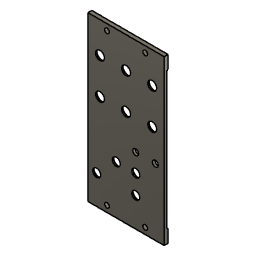
CHORDS Module Faceplate Generator (Autodesk Fusion 360 design; units mm, degrees)
Autodesk Fusion 360 part; units mm, degrees
note: some values were not read from the file. Chosen so that the rebuilt part matches the saved one: which face or edge a step refers to. Set by a fixed rule: which sketch regions a step uses.
(part 1 of 2)
sketch "Sketch2" plane through (0, 0, 0) normal (0, 0, 1) x (1, 0, 0)
  line L0 (29.9, 50) -> (-29.9, 50)
  line L1 (-29.9, 50) -> (-29.9, -50)
  line L2 (-29.9, -50) -> (29.9, -50)
  line L3 (29.9, -50) -> (29.9, 50)
  line L4 (29.9, 50) -> (-29.9, -50) construction
  line L5 (-29.9, 50) -> (29.9, -50) construction
  circle A0 centre (-20.5, 44) radius 4 construction
  circle A1 centre (0, 44) radius 4 construction
  circle A2 centre (20.5, 44) radius 4 construction
  circle A3 centre (-20.5, 16) radius 4 construction
  circle A4 centre (0, 16) radius 4 construction
  circle A5 centre (20.5, 16) radius 4 construction
  circle A6 centre (7.5858, -21.8615) radius 4 construction
  circle A7 centre (22.8605, -21.6215) radius 4 construction
  circle A8 centre (-23.0435, -21.8245) radius 4 construction
  circle A9 centre (-7.6771, -21.8488) radius 4 construction
  circle A10 centre (-23.0823, -36.9623) radius 4 construction
  circle A11 centre (-7.7159, -36.9866) radius 4 construction
  circle A12 centre (7.547, -36.9993) radius 4 construction
  circle A13 centre (22.8217, -36.7594) radius 4 construction
  line L6 (29.9, 50) -> (-29.9, 50)
  line L7 (29.9, -50) -> (-29.9, -50)
  line L8 (-29.9, -50) -> (-29.9, -59.9)
  line L9 (-29.9, -59.9) -> (29.9, -59.9)
  line L10 (29.9, -59.9) -> (29.9, -50)
  circle A14 centre (22.9516, -7.7584) radius 3 construction
  circle A15 centre (7.5143, -7.6767) radius 3 construction
  circle A16 centre (20.5, 16) radius 3.5
  circle A17 centre (20.5, 44) radius 3.5
  circle A18 centre (0, 44) radius 3.5
  circle A19 centre (-20.5, 44) radius 3.5
  circle A20 centre (-20.5, 16) radius 3.5
  circle A21 centre (0, 16) radius 3.5
  line L11 (29.9, 50) -> (-29.9, 50)
  line L12 (-29.9, 50) -> (-29.9, 68.4)
  line L13 (-29.9, 68.4) -> (29.9, 68.4)
  line L14 (29.9, 68.4) -> (29.9, 50)
  circle A22 centre (22.8605, -21.6215) radius 3.15
  circle A23 through (7.5858, -18.7115, 0) (7.5858, -23.4365, 2.728) (7.5858, -23.4365, -2.728) construction
  circle A24 centre (7.5858, -21.8615) radius 3.15
  circle A25 centre (-7.6771, -21.8488) radius 3.15
  circle A26 centre (-23.0435, -21.8245) radius 3.15
  circle A27 centre (22.8217, -36.7594) radius 3.15
  circle A28 centre (7.547, -36.9993) radius 3.15
  circle A29 centre (-7.7159, -36.9866) radius 3.15
  circle A30 centre (-23.0823, -36.9623) radius 3.15
  circle A31 centre (22.9516, -7.7584) radius 2.325
  circle A32 centre (7.5143, -7.6767) radius 2.325
  line L15 (0, 12.5) -> (0, 9.3) construction
  line L16 (0, 9.3) -> (-29.9, 9.3) construction
  line L17 (0, 9.3) -> (29.9, 9.3) construction
  line L18 (0, 9.3) -> (-1, 9.3) construction
  line L19 (-1, 9.3) -> (1, 9.3)
  line L20 (1, 9.3) -> (1, 11.3)
  line L21 (1, 11.3) -> (-1, 11.3)
  line L22 (-1, 11.3) -> (-1, 9.3)
  line L23 (0, 40.5) -> (0, 37.3) construction
  line L24 (0, 37.3) -> (-29.9, 37.3) construction
  line L25 (0, 37.3) -> (29.9, 37.3) construction
  line L26 (0, 37.3) -> (-1, 37.3) construction
  line L27 (-1, 37.3) -> (1, 37.3)
  line L28 (1, 37.3) -> (1, 39.3)
  line L29 (1, 39.3) -> (-1, 39.3)
  line L30 (-1, 39.3) -> (-1, 37.3)
  line L31 (20.5, 44) -> (20.5, 9.3) construction
  line L32 (20.5, 37.3) -> (19.5, 37.3) construction
  line L33 (19.5, 37.3) -> (19.5, 9.3) construction
  line L34 (19.5, 9.3) -> (21.5, 9.3)
  line L35 (21.5, 9.3) -> (21.5, 11.3)
  line L36 (21.5, 11.3) -> (19.5, 11.3)
  line L37 (19.5, 11.3) -> (19.5, 9.3)
  line L38 (19.5, 37.3) -> (21.5, 37.3)
  line L39 (21.5, 37.3) -> (21.5, 39.3)
  line L40 (21.5, 39.3) -> (19.5, 39.3)
  line L41 (19.5, 39.3) -> (19.5, 37.3)
  line L42 (-20.5, 44) -> (-20.5, 9.3) construction
  line L43 (-20.5, 37.3) -> (-21.5, 37.3) construction
  line L44 (-21.5, 37.3) -> (-19.5, 37.3)
  line L45 (-19.5, 37.3) -> (-19.5, 39.3)
  line L46 (-19.5, 39.3) -> (-21.5, 39.3)
  line L47 (-21.5, 39.3) -> (-21.5, 37.3)
  line L48 (-21.5, 9.3) -> (-19.5, 9.3)
  line L49 (-19.5, 9.3) -> (-19.5, 11.3)
  line L50 (-19.5, 11.3) -> (-21.5, 11.3)
  line L51 (-21.5, 11.3) -> (-21.5, 9.3)
  dimension "d1" = 59.8
  dimension "d2" = 100
  dimension "d3" = 8
  dimension "d4" = 8
  dimension "d5" = 8
  dimension "d6" = 8
  dimension "d7" = 8
  dimension "d8" = 8
  dimension "d9" = 8
  dimension "d10" = 8
  dimension "d11" = 8
  dimension "d12" = 8
  dimension "d13" = 8
  dimension "d14" = 8
  dimension "d15" = 8
  dimension "d16" = 8
  dimension "d18" = 9.9
  dimension "d25" = 6
  dimension "d26" = 6
  dimension "d29" = 7
  dimension "d30" = 7
  dimension "d31" = 7
  dimension "d32" = 7
  dimension "d33" = 7
  dimension "d34" = 7
  dimension "d36" = 18.4
  dimension "d37" = 6.3
  dimension "d38" = 6.3
  dimension "d39" = 6.3
  dimension "d40" = 6.3
  dimension "d41" = 6.3
  dimension "d42" = 6.3
  dimension "d43" = 6.3
  dimension "d44" = 6.3
  dimension "d45" = 6.3
  dimension "d47" = 4.65
  dimension "d48" = 4.65
  dimension "d56" = 3.2
  dimension "d57" = 1
  dimension "d58" = 2
  dimension "d59" = 2
  dimension "d60" = 3.2
  dimension "d61" = 1
  dimension "d62" = 2
  dimension "d63" = 2
  dimension "d64" = 1
  dimension "d65" = 2
  dimension "d66" = 2
  dimension "d67" = 2
  dimension "d68" = 2
  dimension "d69" = 1
  dimension "d70" = 2
  dimension "d71" = 2
  dimension "d72" = 2
  dimension "d73" = 2
  constraint horizontal L0
  constraint perpendicular L0 L1
  constraint parallel L0 L2
  constraint parallel L1 L3
  constraint coincident L4 origin
  constraint coincident L5 origin
  constraint horizontal L6
  constraint horizontal L7
  constraint vertical L8
  constraint horizontal L9
  constraint vertical L10
  constraint concentric A5 A16
  constraint concentric A2 A17
  constraint concentric A1 A18
  constraint concentric A0 A19
  constraint concentric A3 A20
  constraint concentric A4 A21
  constraint horizontal L11
  constraint vertical L12
  constraint horizontal L13
  constraint vertical L14
  constraint concentric A7 A22
  constraint concentric A6 A24
  constraint concentric A9 A25
  constraint concentric A8 A26
  constraint concentric A13 A27
  constraint concentric A12 A28
  constraint concentric A11 A29
  constraint concentric A10 A30
  constraint concentric A14 A31
  constraint concentric A15 A32
  constraint coincident A21 L15.start
  constraint vertical L15
  constraint coincident L1 L16.end
  constraint perpendicular L1 L16
  constraint coincident L3 L17.end
  constraint perpendicular L3 L17
  constraint perpendicular L15 L18
  constraint horizontal L19
  constraint vertical L20
  constraint horizontal L21
  constraint vertical L22
  constraint coincident A18 L23.start
  constraint vertical L23
  constraint coincident L1 L24.end
  constraint perpendicular L1 L24
  constraint coincident L3 L25.end
  constraint perpendicular L3 L25
  constraint perpendicular L23 L26
  constraint horizontal L27
  constraint vertical L28
  constraint horizontal L29
  constraint vertical L30
  constraint coincident A2.centre A17.centre
  constraint coincident L17 L31.end
  constraint perpendicular L17 L31
  constraint coincident L31 L32.start
  constraint coincident L25 L32.start
  constraint coincident L25 L32.end
  constraint coincident L17 L33.end
  constraint perpendicular L17 L33
  constraint horizontal L34
  constraint vertical L35
  constraint horizontal L36
  constraint vertical L37
  constraint horizontal L38
  constraint vertical L39
  constraint horizontal L40
  constraint vertical L41
  constraint coincident A0.centre A19.centre
  constraint coincident L16 L42.end
  constraint perpendicular L16 L42
  constraint coincident L24 L43.start
  constraint coincident L42 L43.start
  constraint perpendicular L42 L43
  constraint horizontal L44
  constraint vertical L45
  constraint horizontal L46
  constraint vertical L47
  constraint horizontal L48
  constraint vertical L49
  constraint horizontal L50
  constraint vertical L51
  constraint coincident L16 L48.start
  constraint coincident L1.end L2.start
  constraint coincident L0.end L12
  constraint coincident L0.end L1.start
  measures "d1" distance of L1.end L2.end
  measures "d2" distance of L0.end L1.end
  measures "d3" diameter of A0
  measures "d4" diameter of A1
  measures "d5" diameter of A2
  measures "d6" diameter of A3
  measures "d7" diameter of A4
  measures "d8" diameter of A5
  measures "d9" diameter of A6
  measures "d10" diameter of A7
  measures "d11" diameter of A8
  measures "d12" diameter of A9
  measures "d13" diameter of A12
  measures "d14" diameter of A13
  measures "d15" diameter of A10
  measures "d16" diameter of A11
  measures "d18" distance of L2.end L9.end
  measures "d25" diameter of A14
  measures "d26" diameter of A15
  measures "d29" diameter of A16
  measures "d30" diameter of A17
  measures "d31" diameter of A18
  measures "d32" diameter of A19
  measures "d33" diameter of A20
  measures "d34" diameter of A21
  measures "d36" distance of L0.start L13.end
  measures "d37" diameter of A22
  measures "d39" diameter of A24
  measures "d40" diameter of A25
  measures "d41" diameter of A26
  measures "d42" diameter of A27
  measures "d43" diameter of A28
  measures "d44" diameter of A29
  measures "d45" diameter of A30
  measures "d47" diameter of A31
  measures "d48" diameter of A32
  measures "d56" distance of L15.start L15.end
  measures "d57" distance of L15.end L18.end
  measures "d58" distance of L18.end L19.end
  measures "d59" distance of L18.end L21.end
  measures "d60" distance of L23.start L23.end
  measures "d61" distance of L23.end L26.end
  measures "d62" distance of L26.end L27.end
  measures "d63" distance of L26.end L29.end
  measures "d64" distance of L32.start L32.end
  measures "d65" distance of L33.end L34.end
  measures "d66" distance of L33.end L36.end
  measures "d67" distance of L32.end L38.end
  measures "d68" distance of L32.end L40.end
  measures "d69" distance of L43.start L43.end
  measures "d70" distance of L43.end L44.end
  measures "d71" distance of L43.end L46.end
  measures "d72" distance of L48.start L48.end
  measures "d73" distance of L48.start L50.end
extrude "Extrude2" add sketch "Sketch2" along normal blind 2 contours L0 L1 L2 L3 L6 L7 L11 | L0 L6 L11 L12 L13 L14 | L2 L7 L8 L9 L10 | A22 | A26 | A27 | A29 | L19 L20 L21 L22 | L27 L28 L29 L30 | L34 L35 L36 L37 | L38 L39 L40 L41 | L44 L45 L46 L47 | L48 L49 L50 L51
extrude "Extrude3" cut sketch "Sketch2" along normal blind 1.2 contours L19 L20 L21 L22 | L27 L28 L29 L30 | L34 L35 L36 L37 | L38 L39 L40 L41 | L44 L45 L46 L47 | L48 L49 L50 L51
chamfer "Chamfer1" distance 1 angle 45 4 edges at (-26.2323, -36.9623, 0) (-10.8271, -21.8488, 0) (4.397, -36.9993, 0) (4.4358, -21.8615, 0)
chamfer "Chamfer2" distance 1 angle 45 6 edges at (17.2369, 45.2657, 0) (17.2369, 17.2657, 0) (-3.2631, 17.2657, 0) (-23.7631, 17.2657, 0) (-23.7631, 45.2657, 0) (-3.2631, 45.2657, 0)
move_face "OffsetFaces3" offset -0.3 6 faces at (20.1667, 37.3, 0.4) (-0.3333, 37.3, 0.4) (-20.8333, 37.3, 0.4) (-20.8333, 9.3, 0.4) (-0.3333, 9.3, 0.4) (20.1667, 9.3, 0.4)
move_face "OffsetFaces4" offset -0.3 6 faces at (20.8333, 39.3, 0.4) (0.3333, 39.3, 0.4) (-20.1667, 39.3, 0.4) (-20.1667, 11.3, 0.4) (0.3333, 11.3, 0.4) (20.8333, 11.3, 0.4)
move_face "OffsetFaces5" offset -0.2 6 faces at (19.5, 37.8667, 0.8) (-1, 37.8667, 0.8) (-21.5, 37.8667, 0.8) (-21.5, 9.8667, 0.8) (-1, 9.8667, 0.8) (19.5, 9.8667, 0.8)
move_face "OffsetFaces6" offset -0.2 6 faces at (21.5, 38.7333, 0.8) (21.5, 9.8667, 0.4) (1, 9.8667, 0.4) (1, 37.8667, 0.4) (-19.5, 37.8667, 0.4) (-19.5, 9.8667, 0.4)
move_face "OffsetFaces7" offset 0.5 2 faces at (9.8364, -7.5608, 0.6667) (25.2737, -7.6425, 0.6667)
sketch "Sketch5" plane through (0, 0, 2) normal (0, 0, 1) x (1, 0, 0)
  circle A0 centre (7.5858, -21.8615) radius 3.15
  circle A1 centre (-7.6771, -21.8488) radius 3.15
  circle A2 centre (22.9516, -7.7584) radius 1.825
  circle A3 centre (7.5143, -7.6767) radius 1.825
  line L0 (-29.9, 68.4) -> (-29.9, -59.9)
  line L1 (-29.9, -59.9) -> (29.9, -59.9)
  line L2 (29.9, -59.9) -> (29.9, 68.4)
  line L3 (29.9, 68.4) -> (-29.9, 68.4)
  line L4 (0, 68.4) -> (0, 63.5) construction
  line L5 (15, 68.4) -> (-15, 68.4) construction
  line L6 (-15, 68.4) -> (-15, 58.6) construction
  line L7 (-15, 58.6) -> (15, 58.6) construction
  line L8 (15, 58.6) -> (15, 68.4) construction
  line L9 (15, 68.4) -> (-15, 58.6) construction
  line L10 (-15, 68.4) -> (15, 58.6) construction
  line L11 (0, -59.9) -> (0, -55) construction
  line L12 (15, -50) -> (-15, -50) construction
  line L13 (-15, -50) -> (-15, -60) construction
  line L14 (-15, -60) -> (15, -60) construction
  line L15 (15, -60) -> (15, -50) construction
  line L16 (15, -50) -> (-15, -60) construction
  line L17 (-15, -50) -> (15, -60) construction
  circle A4 centre (-15, -55) radius 1.85
  circle A5 centre (15, -55) radius 1.85
  circle A6 centre (15, 63.5) radius 1.85
  circle A7 centre (-15, 63.5) radius 1.85
  line L18 (0, 44) -> (0, 59) construction
  line L19 (-29.9, -59.9) -> (30, -59.9)
  line L20 (30, -59.9) -> (30, -50)
  line L21 (30, -50) -> (-29.9, -50)
  line L22 (-29.9, -50) -> (-29.9, -59.9)
  line L23 (-29.9, 68.4) -> (29.9, 68.4)
  line L24 (29.9, 68.4) -> (29.9, 58.5)
  line L25 (29.9, 58.5) -> (-29.9, 58.5)
  line L26 (-29.9, 58.5) -> (-29.9, 68.4)
  circle A8 centre (0, 16) radius 3.5
  circle A9 centre (7.547, -36.9993) radius 3.15
  circle A10 centre (20.5, 44) radius 3.5
  circle A11 centre (-20.5, 16) radius 3.5
  circle A12 centre (-23.0823, -36.9623) radius 3.15
  circle A13 centre (-20.5, 44) radius 3.5
  circle A14 centre (0, 44) radius 3.5
  circle A15 centre (20.5, 16) radius 3.5
  point P0 (0, 63.5)
  point P1 (0, -55)
  dimension "d118" = 4.9
  dimension "d119" = 30
  dimension "d120" = 4.9
  dimension "d121" = 30
  dimension "d122" = 10
  dimension "d123" = 3.7
  dimension "d124" = 3.7
  dimension "d125" = 3.7
  dimension "d126" = 3.7
  dimension "d150" = 9.9
  dimension "d151" = 9.9
  constraint midpoint L3 L4.start
  constraint perpendicular L3 L4
  constraint horizontal L5
  constraint perpendicular L5 L6
  constraint parallel L5 L7
  constraint parallel L6 L8
  constraint coincident L9 P0
  constraint coincident L10 P0
  constraint coincident L3 L5.start
  constraint coincident P0 L4.end
  constraint midpoint L1 L11.start
  constraint perpendicular L1 L11
  constraint horizontal L12
  constraint perpendicular L12 L13
  constraint parallel L12 L14
  constraint parallel L13 L15
  constraint coincident L16 P1
  constraint coincident L17 P1
  constraint coincident P1 L11.end
  constraint midpoint L13 A4.centre
  constraint midpoint L15 A5.centre
  constraint midpoint L8 A6.centre
  constraint midpoint L6 A7.centre
  constraint perpendicular L7 L18
  constraint horizontal L19
  constraint vertical L20
  constraint horizontal L21
  constraint vertical L22
  constraint coincident L0.end L1.start
  constraint horizontal L23
  constraint vertical L24
  constraint horizontal L25
  constraint vertical L26
  constraint coincident L2 L24.end
  constraint coincident L0.start L3.end
  measures "d118" distance of L4.start P0
  measures "d119" distance of L6.end L7.end
  measures "d120" distance of L11.start P1
  measures "d121" distance of L13.end L14.end
  measures "d122" distance of L12.end L13.end
  measures "d123" diameter of A4
  measures "d124" diameter of A5
  measures "d125" diameter of A6
  measures "d126" diameter of A7
  measures "d150" distance of L0.end L21.end
  measures "d151" distance of L0.start L25.end
extrude "Extrude9" cut sketch "Sketch5" against normal blind 15 contours A4 | A5 | A6 | A7
sketch "Sketch6" plane through (0, 0, 0) normal (0, 0, -1) x (-1, 0, 0)
  circle A0 centre (15, 63.5) radius 1.85
  circle A1 centre (15, -55) radius 1.85
  circle A2 centre (-15, 63.5) radius 1.85
  circle A3 centre (-15, -55) radius 1.85
  line L0 (1.2, 39.6) -> (1.2, 37)
  line L1 (1.2, 37) -> (-1.2, 37)
  line L2 (-1.2, 37) -> (-1.2, 39.6)
  line L3 (21.7, 11.6) -> (21.7, 9)
  line L4 (21.7, 9) -> (19.3, 9)
  line L5 (19.3, 9) -> (19.3, 11.6)
  line L6 (1.2, 11.6) -> (1.2, 9)
  line L7 (1.2, 9) -> (-1.2, 9)
  line L8 (-1.2, 9) -> (-1.2, 11.6)
  line L9 (-19.3, 11.6) -> (-19.3, 9)
  line L10 (-19.3, 9) -> (-21.7, 9)
  line L11 (-21.7, 9) -> (-21.7, 11.6)
  circle A4 centre (-7.5858, -21.8615) radius 4.15
  line L12 (-19.3, 39.6) -> (-19.3, 37)
  line L13 (-19.3, 37) -> (-21.7, 37)
  line L14 (-21.7, 37) -> (-21.7, 39.6)
  line L15 (21.7, 39.6) -> (21.7, 37)
  line L16 (21.7, 37) -> (19.3, 37)
  line L17 (19.3, 37) -> (19.3, 39.6)
  circle A5 centre (-7.5143, -7.6767) radius 1.825
  circle A6 centre (-22.9516, -7.7584) radius 1.825
  line L18 (-29.9, 68.4) -> (-29.9, -59.9)
  line L19 (-29.9, -59.9) -> (29.9, -59.9)
  line L20 (29.9, -59.9) -> (29.9, 68.4)
  line L21 (29.9, 68.4) -> (-29.9, 68.4)
  circle A7 centre (7.6771, -21.8488) radius 4.15
  spline S0 degree 3 poles (-2.9816, -0.9306) (-2.9816, 1.6475) (-2.9816, 4.2173) (-2.9816, 6.787) knots 0 0 0 0 1 1 1 1
  spline S1 degree 3 poles (-2.9816, 6.787) (6.7641, 6.787) (16.5098, 6.787) (26.2554, 6.787) knots 0 0 0 0 1 1 1 1
  spline S2 degree 3 poles (26.2554, 6.787) (26.2554, -0.5917) (26.2554, -7.9704) (26.2554, -15.3491) knots 0 0 0 0 1 1 1 1
  spline S3 degree 3 poles (26.2554, -15.3491) (16.5098, -15.3491) (6.7641, -15.3491) (-2.9816, -15.3491) knots 0 0 0 0 1 1 1 1
  spline S4 degree 3 poles (-2.9816, -15.3491) (-2.9816, -10.5457) (-2.9816, -5.7423) (-2.9816, -0.9306) knots 0 0 0 0 1 1 1 1
  spline S5 degree 3 poles (-1.9398, 6.3703) (-2.147, 6.3703) (-2.3542, 6.3703) (-2.5601, 6.3703) knots 0 0 0 0 1 1 1 1
  spline S6 degree 3 poles (-2.5601, 6.3703) (-2.5601, 3.6593) (-2.5601, 0.9578) (-2.5601, -1.7426) knots 0 0 0 0 1 1 1 1
  spline S7 degree 3 poles (-2.5601, -1.7426) (-1.6708, -1.7426) (-0.7862, -1.7426) (0.105, -1.7426) knots 0 0 0 0 1 1 1 1
  spline S8 degree 3 poles (0.105, -1.7426) (0.105, -0.081) (0.105, 1.5759) (0.105, 3.2395) knots 0 0 0 0 1 1 1 1
  spline S9 degree 3 poles (0.105, 3.2395) (0.4517, 3.2395) (0.7919, 3.2395) (1.1308, 3.2395) knots 0 0 0 0 1 1 1 1
  spline S10 degree 3 poles (1.1308, 3.2395) (1.1308, 4.2863) (1.1308, 5.3265) (1.1308, 6.3703) knots 0 0 0 0 1 1 1 1
  spline S11 degree 3 poles (1.1308, 6.3703) (0.1096, 6.3703) (-0.9067, 6.3703) (-1.9398, 6.3703) knots 0 0 0 0 1 1 1 1
  spline S12 degree 3 poles (23.1717, -11.4403) (23.1717, -11.5586) (23.1717, -11.6769) (23.1717, -11.8017) knots 0 0 0 0 1 1 1 1
  spline S13 degree 3 poles (23.1717, -11.8017) (22.822, -11.8017) (22.4818, -11.8017) (22.1431, -11.8017) knots 0 0 0 0 1 1 1 1
  spline S14 degree 3 poles (22.1431, -11.8017) (22.1431, -12.8485) (22.1431, -13.8887) (22.1431, -14.9275) knots 0 0 0 0 1 1 1 1
  spline S15 degree 3 poles (22.1431, -14.9275) (23.3771, -14.9275) (24.6062, -14.9275) (25.8339, -14.9275) knots 0 0 0 0 1 1 1 1
  spline S16 degree 3 poles (25.8339, -14.9275) (25.8339, -12.2212) (25.8339, -9.5197) (25.8339, -6.8195) knots 0 0 0 0 1 1 1 1
  spline S17 degree 3 poles (25.8339, -6.8195) (24.9445, -6.8195) (24.0599, -6.8195) (23.1717, -6.8195) knots 0 0 0 0 1 1 1 1
  spline S18 degree 3 poles (23.1717, -6.8195) (23.1717, -8.3574) (23.1717, -9.8905) (23.1717, -11.4403) knots 0 0 0 0 1 1 1 1
  spline S19 degree 3 poles (10.2451, -6.8147) (10.0934, -6.8147) (9.9418, -6.8147) (9.7914, -6.8147) knots 0 0 0 0 1 1 1 1
  spline S20 degree 3 poles (9.7914, -6.8147) (9.7914, -9.5257) (9.7914, -12.2272) (9.7914, -14.9276) knots 0 0 0 0 1 1 1 1
  spline S21 degree 3 poles (9.7914, -14.9276) (11.0252, -14.9276) (12.2543, -14.9276) (13.4824, -14.9276) knots 0 0 0 0 1 1 1 1
  spline S22 degree 3 poles (13.4824, -14.9276) (13.4824, -13.8827) (13.4824, -12.8425) (13.4824, -11.7957) knots 0 0 0 0 1 1 1 1
  spline S23 degree 3 poles (13.4824, -11.7957) (13.1375, -11.7957) (12.7974, -11.7957) (12.4507, -11.7957) knots 0 0 0 0 1 1 1 1
  spline S24 degree 3 poles (12.4507, -11.7957) (12.4507, -10.1321) (12.4507, -8.4752) (12.4507, -6.8147) knots 0 0 0 0 1 1 1 1
  spline S25 degree 3 poles (12.4507, -6.8147) (11.7167, -6.8147) (10.9892, -6.8147) (10.2451, -6.8147) knots 0 0 0 0 1 1 1 1
  spline S26 degree 3 poles (6.6613, -14.9324) (7.563, -14.9324) (8.4646, -14.9324) (9.3653, -14.9324) knots 0 0 0 0 1 1 1 1
  spline S27 degree 3 poles (9.3653, -14.9324) (9.3653, -12.2214) (9.3653, -9.52) (9.3653, -6.8194) knots 0 0 0 0 1 1 1 1
  spline S28 degree 3 poles (9.3653, -6.8194) (8.476, -6.8194) (7.5914, -6.8194) (6.7002, -6.8194) knots 0 0 0 0 1 1 1 1
  spline S29 degree 3 poles (6.7002, -6.8194) (6.7002, -8.481) (6.7002, -10.1379) (6.7002, -11.8015) knots 0 0 0 0 1 1 1 1
  spline S30 degree 3 poles (6.7002, -11.8015) (6.3535, -11.8015) (6.0133, -11.8015) (5.6743, -11.8015) knots 0 0 0 0 1 1 1 1
  spline S31 degree 3 poles (5.6743, -11.8015) (5.6743, -12.8483) (5.6743, -13.8885) (5.6743, -14.9324) knots 0 0 0 0 1 1 1 1
  spline S32 degree 3 poles (5.6743, -14.9324) (6.0009, -14.9324) (6.3228, -14.9324) (6.6613, -14.9324) knots 0 0 0 0 1 1 1 1
  spline S33 degree 3 poles (-2.5648, -10.4235) (-2.5648, -11.9252) (-2.5648, -13.4269) (-2.5648, -14.9276) knots 0 0 0 0 1 1 1 1
  spline S34 degree 3 poles (-2.5648, -14.9276) (-1.3263, -14.9276) (-0.0972, -14.9276) (1.1309, -14.9276) knots 0 0 0 0 1 1 1 1
  spline S35 degree 3 poles (1.1309, -14.9276) (1.1309, -13.8827) (1.1309, -12.8425) (1.1309, -11.7957) knots 0 0 0 0 1 1 1 1
  spline S36 degree 3 poles (1.1309, -11.7957) (0.786, -11.7957) (0.4458, -11.7957) (0.0992, -11.7957) knots 0 0 0 0 1 1 1 1
  spline S37 degree 3 poles (0.0992, -11.7957) (0.0992, -10.1321) (0.0992, -8.4752) (0.0992, -6.8195) knots 0 0 0 0 1 1 1 1
  spline S38 degree 3 poles (0.0992, -6.8195) (-0.792, -6.8195) (-1.6767, -6.8195) (-2.5648, -6.8195) knots 0 0 0 0 1 1 1 1
  spline S39 degree 3 poles (-2.5648, -6.8195) (-2.5648, -8.0185) (-2.5648, -9.2126) (-2.5648, -10.4235) knots 0 0 0 0 1 1 1 1
  spline S40 degree 3 poles (25.8387, -1.6703) (25.8387, 1.0091) (25.8387, 3.6885) (25.8387, 6.3648) knots 0 0 0 0 1 1 1 1
  spline S41 degree 3 poles (25.8387, 6.3648) (24.5987, 6.3648) (23.3696, 6.3648) (22.1438, 6.3648) knots 0 0 0 0 1 1 1 1
  spline S42 degree 3 poles (22.1438, 6.3648) (22.1438, 5.3191) (22.1438, 4.2789) (22.1438, 3.2321) knots 0 0 0 0 1 1 1 1
  spline S43 degree 3 poles (22.1438, 3.2321) (22.4894, 3.2321) (22.8296, 3.2321) (23.1763, 3.2321) knots 0 0 0 0 1 1 1 1
  spline S44 degree 3 poles (23.1763, 3.2321) (23.1763, 1.5685) (23.1763, -0.0884) (23.1763, -1.7474) knots 0 0 0 0 1 1 1 1
  spline S45 degree 3 poles (23.1763, -1.7474) (24.0495, -1.7474) (24.9161, -1.7469) (25.7827, -1.7486) knots 0 0 0 0 1 1 1 1
  spline S46 degree 3 poles (25.7827, -1.7486) (25.8336, -1.7487) (25.8452, -1.73) (25.8387, -1.6703) knots 0 0 0 0 1 1 1 1
  spline S47 degree 3 poles (9.37, -0.7222) (9.37, 1.6407) (9.37, 4.0035) (9.37, 6.3656) knots 0 0 0 0 1 1 1 1
  spline S48 degree 3 poles (9.37, 6.3656) (8.1315, 6.3656) (6.9024, 6.3656) (5.6742, 6.3656) knots 0 0 0 0 1 1 1 1
  spline S49 degree 3 poles (5.6742, 6.3656) (5.6742, 5.3207) (5.6742, 4.2806) (5.6742, 3.2337) knots 0 0 0 0 1 1 1 1
  spline S50 degree 3 poles (5.6742, 3.2337) (6.019, 3.2337) (6.3592, 3.2337) (6.7059, 3.2337) knots 0 0 0 0 1 1 1 1
  spline S51 degree 3 poles (6.7059, 3.2337) (6.7059, 1.5702) (6.7059, -0.0867) (6.7059, -1.7426) knots 0 0 0 0 1 1 1 1
  spline S52 degree 3 poles (6.7059, -1.7426) (7.5971, -1.7426) (8.4817, -1.7426) (9.37, -1.7426) knots 0 0 0 0 1 1 1 1
  spline S53 degree 3 poles (9.37, -1.7426) (9.37, -1.4049) (9.37, -1.0719) (9.37, -0.7222) knots 0 0 0 0 1 1 1 1
  spline S54 degree 3 poles (12.4537, 0.8613) (12.4537, 1.6518) (12.4537, 2.4424) (12.4537, 3.2396) knots 0 0 0 0 1 1 1 1
  spline S55 degree 3 poles (12.4537, 3.2396) (12.8033, 3.2396) (13.1435, 3.2396) (13.4823, 3.2396) knots 0 0 0 0 1 1 1 1
  spline S56 degree 3 poles (13.4823, 3.2396) (13.4823, 4.2864) (13.4823, 5.3266) (13.4823, 6.3655) knots 0 0 0 0 1 1 1 1
  spline S57 degree 3 poles (13.4823, 6.3655) (12.2484, 6.3655) (11.0193, 6.3655) (9.7915, 6.3655) knots 0 0 0 0 1 1 1 1
  spline S58 degree 3 poles (9.7915, 6.3655) (9.7915, 3.6592) (9.7915, 0.9577) (9.7915, -1.7426) knots 0 0 0 0 1 1 1 1
  spline S59 degree 3 poles (9.7915, -1.7426) (10.6808, -1.7426) (11.5655, -1.7426) (12.4537, -1.7426) knots 0 0 0 0 1 1 1 1
  spline S60 degree 3 poles (12.4537, -1.7426) (12.4537, -0.877) (12.4537, -0.0162) (12.4537, 0.8613) knots 0 0 0 0 1 1 1 1
  spline S61 degree 3 poles (5.2528, 6.3257) (5.2586, 6.3996) (5.2016, 6.369) (5.1722, 6.369) knots 0 0 0 0 1 1 1 1
  spline S62 degree 3 poles (5.1722, 6.369) (3.9888, 6.3705) (2.8054, 6.3703) (1.622, 6.3703) knots 0 0 0 0 1 1 1 1
  spline S63 degree 3 poles (1.622, 6.3703) (1.6006, 6.3703) (1.5793, 6.3703) (1.5561, 6.3703) knots 0 0 0 0 1 1 1 1
  spline S64 degree 3 poles (1.5561, 6.3703) (1.5561, 5.3226) (1.5561, 4.2824) (1.5561, 3.2356) knots 0 0 0 0 1 1 1 1
  spline S65 degree 3 poles (1.5561, 3.2356) (1.9, 3.2356) (2.2402, 3.2356) (2.5869, 3.2356) knots 0 0 0 0 1 1 1 1
  spline S66 degree 3 poles (2.5869, 3.2356) (2.5869, 1.572) (2.5869, -0.0849) (2.5869, -1.7435) knots 0 0 0 0 1 1 1 1
  spline S67 degree 3 poles (2.5869, -1.7435) (3.1336, -1.7435) (3.6737, -1.7435) (4.2204, -1.7435) knots 0 0 0 0 1 1 1 1
  spline S68 degree 3 poles (4.2204, -1.7435) (4.2204, -0.0827) (4.2204, 1.5742) (4.2204, 3.2377) knots 0 0 0 0 1 1 1 1
  spline S69 degree 3 poles (4.2204, 3.2377) (4.5671, 3.2377) (4.9073, 3.2377) (5.2528, 3.2377) knots 0 0 0 0 1 1 1 1
  spline S70 degree 3 poles (5.2528, 3.2377) (5.2528, 4.2661) (5.2528, 5.2877) (5.2528, 6.3257) knots 0 0 0 0 1 1 1 1
  spline S71 degree 3 poles (19.3462, -14.9324) (20.1368, -14.9324) (20.9273, -14.9324) (21.7168, -14.9324) knots 0 0 0 0 1 1 1 1
  spline S72 degree 3 poles (21.7168, -14.9324) (21.7168, -13.8827) (21.7168, -12.8425) (21.7168, -11.7957) knots 0 0 0 0 1 1 1 1
  spline S73 degree 3 poles (21.7168, -11.7957) (21.3719, -11.7957) (21.0317, -11.7957) (20.6851, -11.7957) knots 0 0 0 0 1 1 1 1
  spline S74 degree 3 poles (20.6851, -11.7957) (20.6851, -10.1322) (20.6851, -8.4753) (20.6851, -6.8195) knots 0 0 0 0 1 1 1 1
  spline S75 degree 3 poles (20.6851, -6.8195) (20.1384, -6.8195) (19.5983, -6.8195) (19.0516, -6.8195) knots 0 0 0 0 1 1 1 1
  spline S76 degree 3 poles (19.0516, -6.8195) (19.0516, -8.4811) (19.0516, -10.138) (19.0516, -11.8015) knots 0 0 0 0 1 1 1 1
  spline S77 degree 3 poles (19.0516, -11.8015) (18.7049, -11.8015) (18.3648, -11.8015) (18.0258, -11.8015) knots 0 0 0 0 1 1 1 1
  spline S78 degree 3 poles (18.0258, -11.8015) (18.0258, -12.8484) (18.0258, -13.8885) (18.0258, -14.9324) knots 0 0 0 0 1 1 1 1
  spline S79 degree 3 poles (18.0258, -14.9324) (18.4636, -14.9324) (18.8966, -14.9324) (19.3462, -14.9324) knots 0 0 0 0 1 1 1 1
  spline S80 degree 3 poles (16.0958, -14.9324) (16.5975, -14.9324) (17.0991, -14.9324) (17.5996, -14.9324) knots 0 0 0 0 1 1 1 1
  spline S81 degree 3 poles (17.5996, -14.9324) (17.5996, -13.8826) (17.5996, -12.8425) (17.5996, -11.7956) knots 0 0 0 0 1 1 1 1
  spline S82 degree 3 poles (17.5996, -11.7956) (17.2547, -11.7956) (16.9145, -11.7956) (16.5679, -11.7956) knots 0 0 0 0 1 1 1 1
  spline S83 degree 3 poles (16.5679, -11.7956) (16.5679, -10.1321) (16.5679, -8.4752) (16.5679, -6.8195) knots 0 0 0 0 1 1 1 1
  spline S84 degree 3 poles (16.5679, -6.8195) (16.0212, -6.8195) (15.4811, -6.8195) (14.9344, -6.8195) knots 0 0 0 0 1 1 1 1
  spline S85 degree 3 poles (14.9344, -6.8195) (14.9344, -8.4812) (14.9344, -10.1381) (14.9344, -11.8016) knots 0 0 0 0 1 1 1 1
  spline S86 degree 3 poles (14.9344, -11.8016) (14.5877, -11.8016) (14.2476, -11.8016) (13.9087, -11.8016) knots 0 0 0 0 1 1 1 1
  spline S87 degree 3 poles (13.9087, -11.8016) (13.9087, -12.8484) (13.9087, -13.8886) (13.9087, -14.9324) knots 0 0 0 0 1 1 1 1
  spline S88 degree 3 poles (13.9087, -14.9324) (14.6354, -14.9324) (15.3573, -14.9324) (16.0958, -14.9324) knots 0 0 0 0 1 1 1 1
  spline S89 degree 3 poles (5.2528, -14.524) (5.2528, -13.6168) (5.2528, -12.7095) (5.2528, -11.7957) knots 0 0 0 0 1 1 1 1
  spline S90 degree 3 poles (5.2528, -11.7957) (4.9032, -11.7957) (4.563, -11.7957) (4.2164, -11.7957) knots 0 0 0 0 1 1 1 1
  spline S91 degree 3 poles (4.2164, -11.7957) (4.2164, -10.1322) (4.2164, -8.4753) (4.2164, -6.8195) knots 0 0 0 0 1 1 1 1
  spline S92 degree 3 poles (4.2164, -6.8195) (3.6697, -6.8195) (3.1296, -6.8195) (2.5829, -6.8195) knots 0 0 0 0 1 1 1 1
  spline S93 degree 3 poles (2.5829, -6.8195) (2.5829, -8.4811) (2.5829, -10.138) (2.5829, -11.8015) knots 0 0 0 0 1 1 1 1
  spline S94 degree 3 poles (2.5829, -11.8015) (2.2362, -11.8015) (1.8961, -11.8015) (1.5571, -11.8015) knots 0 0 0 0 1 1 1 1
  spline S95 degree 3 poles (1.5571, -11.8015) (1.5571, -12.8484) (1.5571, -13.8885) (1.5571, -14.9276) knots 0 0 0 0 1 1 1 1
  spline S96 degree 3 poles (1.5571, -14.9276) (2.7909, -14.9276) (4.02, -14.9276) (5.2528, -14.9276) knots 0 0 0 0 1 1 1 1
  spline S97 degree 3 poles (5.2528, -14.9276) (5.2528, -14.7955) (5.2528, -14.6681) (5.2528, -14.524) knots 0 0 0 0 1 1 1 1
  spline S98 degree 3 poles (19.0545, 0.978) (19.0545, 0.0708) (19.0545, -0.8365) (19.0545, -1.7426) knots 0 0 0 0 1 1 1 1
  spline S99 degree 3 poles (19.0545, -1.7426) (19.6042, -1.7426) (20.1443, -1.7426) (20.6909, -1.7426) knots 0 0 0 0 1 1 1 1
  spline S100 degree 3 poles (20.6909, -1.7426) (20.6909, -0.0809) (20.6909, 1.576) (20.6909, 3.2395) knots 0 0 0 0 1 1 1 1
  spline S101 degree 3 poles (20.6909, 3.2395) (21.0376, 3.2395) (21.3778, 3.2395) (21.7167, 3.2395) knots 0 0 0 0 1 1 1 1
  spline S102 degree 3 poles (21.7167, 3.2395) (21.7167, 4.2863) (21.7167, 5.3265) (21.7167, 6.3655) knots 0 0 0 0 1 1 1 1
  spline S103 degree 3 poles (21.7167, 6.3655) (20.4829, 6.3655) (19.2538, 6.3655) (18.0258, 6.3655) knots 0 0 0 0 1 1 1 1
  spline S104 degree 3 poles (18.0258, 6.3655) (18.0258, 5.3206) (18.0258, 4.2805) (18.0258, 3.2336) knots 0 0 0 0 1 1 1 1
  spline S105 degree 3 poles (18.0258, 3.2336) (18.3707, 3.2336) (18.7109, 3.2336) (19.0545, 3.2336) knots 0 0 0 0 1 1 1 1
  spline S106 degree 3 poles (19.0545, 3.2336) (19.0545, 2.4829) (19.0545, 1.7388) (19.0545, 0.978) knots 0 0 0 0 1 1 1 1
  spline S107 degree 3 poles (16.5709, -0.0888) (16.5709, 1.0184) (16.5709, 2.1256) (16.5709, 3.2395) knots 0 0 0 0 1 1 1 1
  spline S108 degree 3 poles (16.5709, 3.2395) (16.9204, 3.2395) (17.2606, 3.2395) (17.5996, 3.2395) knots 0 0 0 0 1 1 1 1
  spline S109 degree 3 poles (17.5996, 3.2395) (17.5996, 4.2863) (17.5996, 5.3265) (17.5996, 6.3655) knots 0 0 0 0 1 1 1 1
  spline S110 degree 3 poles (17.5996, 6.3655) (16.3657, 6.3655) (15.1366, 6.3655) (13.9086, 6.3655) knots 0 0 0 0 1 1 1 1
  spline S111 degree 3 poles (13.9086, 6.3655) (13.9086, 5.3206) (13.9086, 4.2805) (13.9086, 3.2336) knots 0 0 0 0 1 1 1 1
  spline S112 degree 3 poles (13.9086, 3.2336) (14.2535, 3.2336) (14.5937, 3.2336) (14.9403, 3.2336) knots 0 0 0 0 1 1 1 1
  spline S113 degree 3 poles (14.9403, 3.2336) (14.9403, 1.5701) (14.9403, -0.0868) (14.9403, -1.7426) knots 0 0 0 0 1 1 1 1
  spline S114 degree 3 poles (14.9403, -1.7426) (15.487, -1.7426) (16.0271, -1.7426) (16.5709, -1.7426) knots 0 0 0 0 1 1 1 1
  spline S115 degree 3 poles (16.5709, -1.7426) (16.5709, -1.1937) (16.5709, -0.6496) (16.5709, -0.0888) knots 0 0 0 0 1 1 1 1
  spline S116 degree 3 poles (19.8803, -5.6985) (19.9781, -5.561) (20.0939, -5.4329) (20.1704, -5.2845) knots 0 0 0 0 1 1 1 1
  spline S117 degree 3 poles (20.1704, -5.2845) (20.439, -4.763) (20.4718, -4.2122) (20.3251, -3.6506) knots 0 0 0 0 1 1 1 1
  spline S118 degree 3 poles (20.3251, -3.6506) (20.1823, -3.104) (19.8492, -2.7066) (19.3445, -2.4547) knots 0 0 0 0 1 1 1 1
  spline S119 degree 3 poles (19.3445, -2.4547) (19.0001, -2.2829) (18.6308, -2.2175) (18.2492, -2.216) knots 0 0 0 0 1 1 1 1
  spline S120 degree 3 poles (18.2492, -2.216) (17.713, -2.2138) (17.1769, -2.2154) (16.6407, -2.2154) knots 0 0 0 0 1 1 1 1
  spline S121 degree 3 poles (16.6407, -2.2154) (16.6194, -2.2154) (16.5981, -2.2154) (16.5762, -2.2154) knots 0 0 0 0 1 1 1 1
  spline S122 degree 3 poles (16.5762, -2.2154) (16.5762, -3.5911) (16.5762, -4.9588) (16.5762, -6.3152) knots 0 0 0 0 1 1 1 1
  spline S123 degree 3 poles (16.5762, -6.3152) (17.2339, -6.3152) (17.8871, -6.3365) (18.5382, -6.3084) knots 0 0 0 0 1 1 1 1
  spline S124 degree 3 poles (18.5382, -6.3084) (19.0512, -6.2863) (19.5057, -6.0811) (19.8803, -5.6985) knots 0 0 0 0 1 1 1 1
  spline S125 degree 3 poles (15.3359, -2.49) (15.0702, -2.2889) (14.7645, -2.2155) (14.4381, -2.2146) knots 0 0 0 0 1 1 1 1
  spline S126 degree 3 poles (14.4381, -2.2146) (13.7992, -2.2129) (13.1604, -2.2141) (12.5215, -2.2142) knots 0 0 0 0 1 1 1 1
  spline S127 degree 3 poles (12.5215, -2.2142) (12.5003, -2.2142) (12.479, -2.2161) (12.4579, -2.2171) knots 0 0 0 0 1 1 1 1
  spline S128 degree 3 poles (12.4579, -2.2171) (12.4579, -3.5907) (12.4579, -4.9586) (12.4579, -6.3271) knots 0 0 0 0 1 1 1 1
  spline S129 degree 3 poles (12.4579, -6.3271) (12.8021, -6.3271) (13.1422, -6.3271) (13.4889, -6.3271) knots 0 0 0 0 1 1 1 1
  spline S130 degree 3 poles (13.4889, -6.3271) (13.4889, -5.8607) (13.4889, -5.3983) (13.4889, -4.9311) knots 0 0 0 0 1 1 1 1
  spline S131 degree 3 poles (13.4889, -4.9311) (13.6421, -4.9311) (13.7889, -4.9347) (13.9354, -4.9294) knots 0 0 0 0 1 1 1 1
  spline S132 degree 3 poles (13.9354, -4.9294) (13.9954, -4.9272) (14.0209, -4.95) (14.0449, -5.001) knots 0 0 0 0 1 1 1 1
  spline S133 degree 3 poles (14.0449, -5.001) (14.2534, -5.4444) (14.4647, -5.8864) (14.675, -6.3286) knots 0 0 0 0 1 1 1 1
  spline S134 degree 3 poles (14.675, -6.3286) (15.0653, -6.3286) (15.4534, -6.3286) (15.8523, -6.3286) knots 0 0 0 0 1 1 1 1
  spline S135 degree 3 poles (15.8523, -6.3286) (15.5798, -5.8213) (15.3108, -5.3205) (15.0414, -4.8191) knots 0 0 0 0 1 1 1 1
  spline S136 degree 3 poles (15.0414, -4.8191) (16.0475, -4.4321) (16.0423, -3.0161) (15.3359, -2.49) knots 0 0 0 0 1 1 1 1
  spline S137 degree 3 poles (8.8209, -6.2891) (9.1938, -6.4143) (9.5752, -6.4451) (9.9625, -6.3817) knots 0 0 0 0 1 1 1 1
  spline S138 degree 3 poles (9.9625, -6.3817) (10.5708, -6.2819) (11.0607, -5.9903) (11.3926, -5.4625) knots 0 0 0 0 1 1 1 1
  spline S139 degree 3 poles (11.3926, -5.4625) (11.6991, -4.975) (11.7777, -4.4385) (11.6844, -3.8784) knots 0 0 0 0 1 1 1 1
  spline S140 degree 3 poles (11.6844, -3.8784) (11.5798, -3.2502) (11.2593, -2.7583) (10.7025, -2.4367) knots 0 0 0 0 1 1 1 1
  spline S141 degree 3 poles (10.7025, -2.4367) (10.2832, -2.1946) (9.8261, -2.1155) (9.3469, -2.1623) knots 0 0 0 0 1 1 1 1
  spline S142 degree 3 poles (9.3469, -2.1623) (8.7507, -2.2206) (8.2477, -2.4633) (7.8763, -2.9414) knots 0 0 0 0 1 1 1 1
  spline S143 degree 3 poles (7.8763, -2.9414) (7.5204, -3.3995) (7.3936, -3.9287) (7.4511, -4.4994) knots 0 0 0 0 1 1 1 1
  spline S144 degree 3 poles (7.4511, -4.4994) (7.5385, -5.3685) (7.9838, -5.9726) (8.8209, -6.2891) knots 0 0 0 0 1 1 1 1
  spline S145 degree 3 poles (4.7777, -3.7476) (4.4928, -3.7476) (4.2079, -3.7476) (3.9166, -3.7476) knots 0 0 0 0 1 1 1 1
  spline S146 degree 3 poles (3.9166, -3.7476) (3.9166, -3.2315) (3.9166, -2.7248) (3.9166, -2.2187) knots 0 0 0 0 1 1 1 1
  spline S147 degree 3 poles (3.9166, -2.2187) (3.57, -2.2187) (3.23, -2.2187) (2.89, -2.2187) knots 0 0 0 0 1 1 1 1
  spline S148 degree 3 poles (2.89, -2.2187) (2.89, -3.5909) (2.89, -4.9586) (2.89, -6.3272) knots 0 0 0 0 1 1 1 1
  spline S149 degree 3 poles (2.89, -6.3272) (3.2342, -6.3272) (3.5742, -6.3272) (3.9202, -6.3272) knots 0 0 0 0 1 1 1 1
  spline S150 degree 3 poles (3.9202, -6.3272) (3.9202, -5.7744) (3.9202, -5.2257) (3.9202, -4.6731) knots 0 0 0 0 1 1 1 1
  spline S151 degree 3 poles (3.9202, -4.6731) (4.4716, -4.6731) (5.0171, -4.6731) (5.5715, -4.6731) knots 0 0 0 0 1 1 1 1
  spline S152 degree 3 poles (5.5715, -4.6731) (5.5715, -5.2277) (5.5715, -5.7784) (5.5715, -6.3259) knots 0 0 0 0 1 1 1 1
  spline S153 degree 3 poles (5.5715, -6.3259) (5.9205, -6.3259) (6.2605, -6.3259) (6.598, -6.3259) knots 0 0 0 0 1 1 1 1
  spline S154 degree 3 poles (6.598, -6.3259) (6.598, -4.9528) (6.598, -3.5851) (6.598, -2.219) knots 0 0 0 0 1 1 1 1
  spline S155 degree 3 poles (6.598, -2.219) (6.2529, -2.219) (5.9128, -2.219) (5.5663, -2.219) knots 0 0 0 0 1 1 1 1
  spline S156 degree 3 poles (5.5663, -2.219) (5.5663, -2.7307) (5.5663, -3.2374) (5.5663, -3.7476) knots 0 0 0 0 1 1 1 1
  spline S157 degree 3 poles (5.5663, -3.7476) (5.3047, -3.7476) (5.0496, -3.7476) (4.7777, -3.7476) knots 0 0 0 0 1 1 1 1
  spline S158 degree 3 poles (22.9254, -6.4106) (23.1349, -6.3728) (23.3522, -6.3587) (23.5524, -6.2929) knots 0 0 0 0 1 1 1 1
  spline S159 degree 3 poles (23.5524, -6.2929) (24.4064, -6.0124) (24.5516, -5.2235) (24.4065, -4.7003) knots 0 0 0 0 1 1 1 1
  spline S160 degree 3 poles (24.4065, -4.7003) (24.316, -4.3737) (24.0819, -4.1733) (23.789, -4.0313) knots 0 0 0 0 1 1 1 1
  spline S161 degree 3 poles (23.789, -4.0313) (23.4844, -3.8837) (23.1543, -3.8216) (22.8281, -3.7446) knots 0 0 0 0 1 1 1 1
  spline S162 degree 3 poles (22.8281, -3.7446) (22.6594, -3.7048) (22.4872, -3.6628) (22.3312, -3.5903) knots 0 0 0 0 1 1 1 1
  spline S163 degree 3 poles (22.3312, -3.5903) (22.1442, -3.5034) (22.1419, -3.2588) (22.3135, -3.1412) knots 0 0 0 0 1 1 1 1
  spline S164 degree 3 poles (22.3135, -3.1412) (22.3516, -3.1151) (22.3965, -3.0955) (22.4411, -3.0831) knots 0 0 0 0 1 1 1 1
  spline S165 degree 3 poles (22.4411, -3.0831) (22.6254, -3.0318) (22.81, -3.0529) (22.9932, -3.0916) knots 0 0 0 0 1 1 1 1
  spline S166 degree 3 poles (22.9932, -3.0916) (23.2915, -3.1547) (23.5573, -3.2871) (23.7958, -3.481) knots 0 0 0 0 1 1 1 1
  spline S167 degree 3 poles (23.7958, -3.481) (23.9841, -3.2265) (24.1702, -2.9751) (24.3582, -2.7211) knots 0 0 0 0 1 1 1 1
  spline S168 degree 3 poles (24.3582, -2.7211) (24.3112, -2.6833) (24.269, -2.6472) (24.2246, -2.6141) knots 0 0 0 0 1 1 1 1
  spline S169 degree 3 poles (24.2246, -2.6141) (23.8053, -2.3004) (23.3266, -2.1652) (22.8099, -2.1493) knots 0 0 0 0 1 1 1 1
  spline S170 degree 3 poles (22.8099, -2.1493) (22.5074, -2.14) (22.2119, -2.1804) (21.9309, -2.2991) knots 0 0 0 0 1 1 1 1
  spline S171 degree 3 poles (21.9309, -2.2991) (21.2975, -2.5667) (20.9904, -3.2162) (21.2023, -3.8388) knots 0 0 0 0 1 1 1 1
  spline S172 degree 3 poles (21.2023, -3.8388) (21.3157, -4.1722) (21.5626, -4.3793) (21.8784, -4.4933) knots 0 0 0 0 1 1 1 1
  spline S173 degree 3 poles (21.8784, -4.4933) (22.1557, -4.5935) (22.4467, -4.6562) (22.7327, -4.7317) knots 0 0 0 0 1 1 1 1
  spline S174 degree 3 poles (22.7327, -4.7317) (22.9173, -4.7803) (23.1088, -4.8095) (23.2715, -4.9181) knots 0 0 0 0 1 1 1 1
  spline S175 degree 3 poles (23.2715, -4.9181) (23.4475, -5.0356) (23.4555, -5.2526) (23.2856, -5.3785) knots 0 0 0 0 1 1 1 1
  spline S176 degree 3 poles (23.2856, -5.3785) (23.2248, -5.4235) (23.1505, -5.4558) (23.0774, -5.4773) knots 0 0 0 0 1 1 1 1
  spline S177 degree 3 poles (23.0774, -5.4773) (22.9146, -5.5251) (22.7472, -5.5135) (22.5817, -5.489) knots 0 0 0 0 1 1 1 1
  spline S178 degree 3 poles (22.5817, -5.489) (22.1842, -5.4301) (21.8467, -5.2515) (21.5574, -4.9629) knots 0 0 0 0 1 1 1 1
  spline S179 degree 3 poles (21.5574, -4.9629) (21.3764, -5.2281) (21.1969, -5.4911) (21.0063, -5.7703) knots 0 0 0 0 1 1 1 1
  spline S180 degree 3 poles (21.0063, -5.7703) (21.1384, -5.8684) (21.263, -5.9751) (21.4008, -6.0606) knots 0 0 0 0 1 1 1 1
  spline S181 degree 3 poles (21.4008, -6.0606) (21.8629, -6.3473) (22.3762, -6.4254) (22.9254, -6.4106) knots 0 0 0 0 1 1 1 1
  spline S182 degree 3 poles (-1.7079, -4.7148) (-1.6474, -5.0416) (-1.5217, -5.3399) (-1.3208, -5.6058) knots 0 0 0 0 1 1 1 1
  spline S183 degree 3 poles (-1.3208, -5.6058) (-0.7701, -6.3349) (0.2175, -6.5625) (1.0233, -6.3208) knots 0 0 0 0 1 1 1 1
  spline S184 degree 3 poles (1.0233, -6.3208) (1.5549, -6.1614) (1.915, -5.8044) (2.1626, -5.3099) knots 0 0 0 0 1 1 1 1
  spline S185 degree 3 poles (2.1626, -5.3099) (1.8643, -5.1642) (1.5722, -5.0215) (1.28, -4.8789) knots 0 0 0 0 1 1 1 1
  spline S186 degree 3 poles (1.28, -4.8789) (1.1014, -5.2458) (0.8181, -5.4624) (0.4124, -5.4753) knots 0 0 0 0 1 1 1 1
  spline S187 degree 3 poles (0.4124, -5.4753) (0.0047, -5.4883) (-0.3165, -5.3059) (-0.5183, -4.9527) knots 0 0 0 0 1 1 1 1
  spline S188 degree 3 poles (-0.5183, -4.9527) (-0.7716, -4.5093) (-0.7704, -4.0506) (-0.5172, -3.6064) knots 0 0 0 0 1 1 1 1
  spline S189 degree 3 poles (-0.5172, -3.6064) (-0.2715, -3.1751) (0.2351, -2.9817) (0.6845, -3.1336) knots 0 0 0 0 1 1 1 1
  spline S190 degree 3 poles (0.6845, -3.1336) (0.9617, -3.2273) (1.1567, -3.415) (1.2783, -3.6842) knots 0 0 0 0 1 1 1 1
  spline S191 degree 3 poles (1.2783, -3.6842) (1.5737, -3.5398) (1.8658, -3.397) (2.1625, -3.252) knots 0 0 0 0 1 1 1 1
  spline S192 degree 3 poles (2.1625, -3.252) (1.9652, -2.8548) (1.6948, -2.5408) (1.2998, -2.3478) knots 0 0 0 0 1 1 1 1
  spline S193 degree 3 poles (1.2998, -2.3478) (0.889, -2.1471) (0.4535, -2.1068) (0.0089, -2.1814) knots 0 0 0 0 1 1 1 1
  spline S194 degree 3 poles (0.0089, -2.1814) (-0.7062, -2.3015) (-1.2408, -2.6758) (-1.5499, -3.342) knots 0 0 0 0 1 1 1 1
  spline S195 degree 3 poles (-1.5499, -3.342) (-1.7511, -3.7755) (-1.7861, -4.2326) (-1.7079, -4.7148) knots 0 0 0 0 1 1 1 1
  spline S196 degree 3 poles (-1.9314, 6.3703) (-0.9067, 6.3703) (0.1096, 6.3703) (1.1308, 6.3703) knots 0 0 0 0 1 1 1 1
  spline S197 degree 3 poles (1.1308, 6.3703) (1.1308, 5.3265) (1.1308, 4.2863) (1.1308, 3.2395) knots 0 0 0 0 1 1 1 1
  spline S198 degree 3 poles (1.1308, 3.2395) (0.7919, 3.2395) (0.4517, 3.2395) (0.105, 3.2395) knots 0 0 0 0 1 1 1 1
  spline S199 degree 3 poles (0.105, 3.2395) (0.105, 1.5759) (0.105, -0.081) (0.105, -1.7426) knots 0 0 0 0 1 1 1 1
  spline S200 degree 3 poles (0.105, -1.7426) (-0.7862, -1.7426) (-1.6708, -1.7426) (-2.5601, -1.7426) knots 0 0 0 0 1 1 1 1
  spline S201 degree 3 poles (-2.5601, -1.7426) (-2.5601, 0.9578) (-2.5601, 3.6593) (-2.5601, 6.3703) knots 0 0 0 0 1 1 1 1
  spline S202 degree 3 poles (-2.5601, 6.3703) (-2.3542, 6.3703) (-2.147, 6.3703) (-1.9314, 6.3703) knots 0 0 0 0 1 1 1 1
  spline S203 degree 3 poles (23.1717, -11.4319) (23.1717, -9.8905) (23.1717, -8.3574) (23.1717, -6.8195) knots 0 0 0 0 1 1 1 1
  spline S204 degree 3 poles (23.1717, -6.8195) (24.0599, -6.8195) (24.9445, -6.8195) (25.8339, -6.8195) knots 0 0 0 0 1 1 1 1
  spline S205 degree 3 poles (25.8339, -6.8195) (25.8339, -9.5197) (25.8339, -12.2212) (25.8339, -14.9275) knots 0 0 0 0 1 1 1 1
  spline S206 degree 3 poles (25.8339, -14.9275) (24.6062, -14.9275) (23.3771, -14.9275) (22.1431, -14.9275) knots 0 0 0 0 1 1 1 1
  spline S207 degree 3 poles (22.1431, -14.9275) (22.1431, -13.8887) (22.1431, -12.8485) (22.1431, -11.8017) knots 0 0 0 0 1 1 1 1
  spline S208 degree 3 poles (22.1431, -11.8017) (22.4818, -11.8017) (22.822, -11.8017) (23.1717, -11.8017) knots 0 0 0 0 1 1 1 1
  spline S209 degree 3 poles (23.1717, -11.8017) (23.1717, -11.6769) (23.1717, -11.5586) (23.1717, -11.4319) knots 0 0 0 0 1 1 1 1
  spline S210 degree 3 poles (10.2534, -6.8147) (10.9892, -6.8147) (11.7167, -6.8147) (12.4507, -6.8147) knots 0 0 0 0 1 1 1 1
  spline S211 degree 3 poles (12.4507, -6.8147) (12.4507, -8.4752) (12.4507, -10.1321) (12.4507, -11.7957) knots 0 0 0 0 1 1 1 1
  spline S212 degree 3 poles (12.4507, -11.7957) (12.7974, -11.7957) (13.1375, -11.7957) (13.4824, -11.7957) knots 0 0 0 0 1 1 1 1
  spline S213 degree 3 poles (13.4824, -11.7957) (13.4824, -12.8425) (13.4824, -13.8827) (13.4824, -14.9276) knots 0 0 0 0 1 1 1 1
  spline S214 degree 3 poles (13.4824, -14.9276) (12.2543, -14.9276) (11.0252, -14.9276) (9.7914, -14.9276) knots 0 0 0 0 1 1 1 1
  spline S215 degree 3 poles (9.7914, -14.9276) (9.7914, -12.2272) (9.7914, -9.5257) (9.7914, -6.8147) knots 0 0 0 0 1 1 1 1
  spline S216 degree 3 poles (9.7914, -6.8147) (9.9418, -6.8147) (10.0934, -6.8147) (10.2534, -6.8147) knots 0 0 0 0 1 1 1 1
  spline S217 degree 3 poles (6.653, -14.9324) (6.3228, -14.9324) (6.0009, -14.9324) (5.6743, -14.9324) knots 0 0 0 0 1 1 1 1
  spline S218 degree 3 poles (5.6743, -14.9324) (5.6743, -13.8885) (5.6743, -12.8483) (5.6743, -11.8015) knots 0 0 0 0 1 1 1 1
  spline S219 degree 3 poles (5.6743, -11.8015) (6.0133, -11.8015) (6.3535, -11.8015) (6.7002, -11.8015) knots 0 0 0 0 1 1 1 1
  spline S220 degree 3 poles (6.7002, -11.8015) (6.7002, -10.1379) (6.7002, -8.481) (6.7002, -6.8194) knots 0 0 0 0 1 1 1 1
  spline S221 degree 3 poles (6.7002, -6.8194) (7.5914, -6.8194) (8.476, -6.8194) (9.3653, -6.8194) knots 0 0 0 0 1 1 1 1
  spline S222 degree 3 poles (9.3653, -6.8194) (9.3653, -9.52) (9.3653, -12.2214) (9.3653, -14.9324) knots 0 0 0 0 1 1 1 1
  spline S223 degree 3 poles (9.3653, -14.9324) (8.4646, -14.9324) (7.563, -14.9324) (6.653, -14.9324) knots 0 0 0 0 1 1 1 1
  spline S224 degree 3 poles (-2.5648, -10.4151) (-2.5648, -9.2126) (-2.5648, -8.0185) (-2.5648, -6.8195) knots 0 0 0 0 1 1 1 1
  spline S225 degree 3 poles (-2.5648, -6.8195) (-1.6767, -6.8195) (-0.792, -6.8195) (0.0992, -6.8195) knots 0 0 0 0 1 1 1 1
  spline S226 degree 3 poles (0.0992, -6.8195) (0.0992, -8.4752) (0.0992, -10.1321) (0.0992, -11.7957) knots 0 0 0 0 1 1 1 1
  spline S227 degree 3 poles (0.0992, -11.7957) (0.4458, -11.7957) (0.786, -11.7957) (1.1309, -11.7957) knots 0 0 0 0 1 1 1 1
  spline S228 degree 3 poles (1.1309, -11.7957) (1.1309, -12.8425) (1.1309, -13.8827) (1.1309, -14.9276) knots 0 0 0 0 1 1 1 1
  spline S229 degree 3 poles (1.1309, -14.9276) (-0.0972, -14.9276) (-1.3263, -14.9276) (-2.5648, -14.9276) knots 0 0 0 0 1 1 1 1
  spline S230 degree 3 poles (-2.5648, -14.9276) (-2.5648, -13.4269) (-2.5648, -11.9252) (-2.5648, -10.4151) knots 0 0 0 0 1 1 1 1
  spline S231 degree 3 poles (25.8387, -1.6784) (25.8452, -1.73) (25.8336, -1.7487) (25.7827, -1.7486) knots 0 0 0 0 1 1 1 1
  spline S232 degree 3 poles (25.7827, -1.7486) (24.9161, -1.7469) (24.0495, -1.7474) (23.1763, -1.7474) knots 0 0 0 0 1 1 1 1
  spline S233 degree 3 poles (23.1763, -1.7474) (23.1763, -0.0884) (23.1763, 1.5685) (23.1763, 3.2321) knots 0 0 0 0 1 1 1 1
  spline S234 degree 3 poles (23.1763, 3.2321) (22.8296, 3.2321) (22.4894, 3.2321) (22.1438, 3.2321) knots 0 0 0 0 1 1 1 1
  spline S235 degree 3 poles (22.1438, 3.2321) (22.1438, 4.2789) (22.1438, 5.3191) (22.1438, 6.3648) knots 0 0 0 0 1 1 1 1
  spline S236 degree 3 poles (22.1438, 6.3648) (23.3696, 6.3648) (24.5987, 6.3648) (25.8387, 6.3648) knots 0 0 0 0 1 1 1 1
  spline S237 degree 3 poles (25.8387, 6.3648) (25.8387, 3.6885) (25.8387, 1.0091) (25.8387, -1.6784) knots 0 0 0 0 1 1 1 1
  spline S238 degree 3 poles (9.37, -0.7306) (9.37, -1.0719) (9.37, -1.4049) (9.37, -1.7426) knots 0 0 0 0 1 1 1 1
  spline S239 degree 3 poles (9.37, -1.7426) (8.4817, -1.7426) (7.5971, -1.7426) (6.7059, -1.7426) knots 0 0 0 0 1 1 1 1
  spline S240 degree 3 poles (6.7059, -1.7426) (6.7059, -0.0867) (6.7059, 1.5702) (6.7059, 3.2337) knots 0 0 0 0 1 1 1 1
  spline S241 degree 3 poles (6.7059, 3.2337) (6.3592, 3.2337) (6.019, 3.2337) (5.6742, 3.2337) knots 0 0 0 0 1 1 1 1
  spline S242 degree 3 poles (5.6742, 3.2337) (5.6742, 4.2806) (5.6742, 5.3207) (5.6742, 6.3656) knots 0 0 0 0 1 1 1 1
  spline S243 degree 3 poles (5.6742, 6.3656) (6.9024, 6.3656) (8.1315, 6.3656) (9.37, 6.3656) knots 0 0 0 0 1 1 1 1
  spline S244 degree 3 poles (9.37, 6.3656) (9.37, 4.0035) (9.37, 1.6407) (9.37, -0.7306) knots 0 0 0 0 1 1 1 1
  spline S245 degree 3 poles (12.4537, 0.8529) (12.4537, -0.0162) (12.4537, -0.877) (12.4537, -1.7426) knots 0 0 0 0 1 1 1 1
  spline S246 degree 3 poles (12.4537, -1.7426) (11.5655, -1.7426) (10.6808, -1.7426) (9.7915, -1.7426) knots 0 0 0 0 1 1 1 1
  spline S247 degree 3 poles (9.7915, -1.7426) (9.7915, 0.9577) (9.7915, 3.6592) (9.7915, 6.3655) knots 0 0 0 0 1 1 1 1
  spline S248 degree 3 poles (9.7915, 6.3655) (11.0193, 6.3655) (12.2484, 6.3655) (13.4823, 6.3655) knots 0 0 0 0 1 1 1 1
  spline S249 degree 3 poles (13.4823, 6.3655) (13.4823, 5.3266) (13.4823, 4.2864) (13.4823, 3.2396) knots 0 0 0 0 1 1 1 1
  spline S250 degree 3 poles (13.4823, 3.2396) (13.1435, 3.2396) (12.8033, 3.2396) (12.4537, 3.2396) knots 0 0 0 0 1 1 1 1
  spline S251 degree 3 poles (12.4537, 3.2396) (12.4537, 2.4424) (12.4537, 1.6518) (12.4537, 0.8529) knots 0 0 0 0 1 1 1 1
  spline S252 degree 3 poles (5.2528, 6.3175) (5.2528, 5.2877) (5.2528, 4.2661) (5.2528, 3.2377) knots 0 0 0 0 1 1 1 1
  spline S253 degree 3 poles (5.2528, 3.2377) (4.9073, 3.2377) (4.5671, 3.2377) (4.2204, 3.2377) knots 0 0 0 0 1 1 1 1
  spline S254 degree 3 poles (4.2204, 3.2377) (4.2204, 1.5742) (4.2204, -0.0827) (4.2204, -1.7435) knots 0 0 0 0 1 1 1 1
  spline S255 degree 3 poles (4.2204, -1.7435) (3.6737, -1.7435) (3.1336, -1.7435) (2.5869, -1.7435) knots 0 0 0 0 1 1 1 1
  spline S256 degree 3 poles (2.5869, -1.7435) (2.5869, -0.0849) (2.5869, 1.572) (2.5869, 3.2356) knots 0 0 0 0 1 1 1 1
  spline S257 degree 3 poles (2.5869, 3.2356) (2.2402, 3.2356) (1.9, 3.2356) (1.5561, 3.2356) knots 0 0 0 0 1 1 1 1
  spline S258 degree 3 poles (1.5561, 3.2356) (1.5561, 4.2824) (1.5561, 5.3226) (1.5561, 6.3703) knots 0 0 0 0 1 1 1 1
  spline S259 degree 3 poles (1.5561, 6.3703) (1.5793, 6.3703) (1.6006, 6.3703) (1.622, 6.3703) knots 0 0 0 0 1 1 1 1
  spline S260 degree 3 poles (1.622, 6.3703) (2.8054, 6.3703) (3.9888, 6.3705) (5.1722, 6.369) knots 0 0 0 0 1 1 1 1
  spline S261 degree 3 poles (5.1722, 6.369) (5.2016, 6.369) (5.2586, 6.3996) (5.2528, 6.3175) knots 0 0 0 0 1 1 1 1